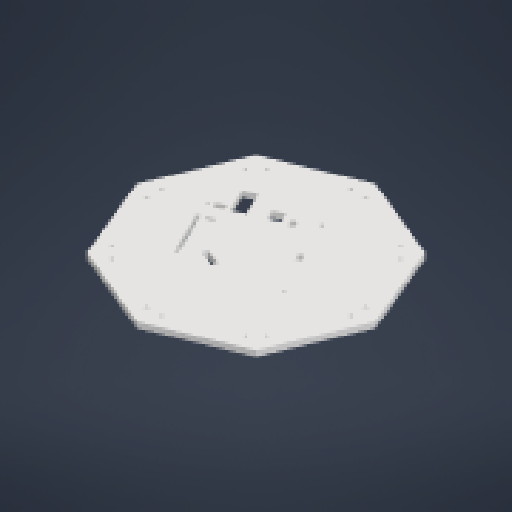
# Autodesk Inventor part: Bund
Saved by Autodesk Inventor 2026.1 (Build 301233020, 233B)
## iProperties
Created: 2026-04-22
Part Number: Bund
Material: Generic
Document SubType Name: Modeling
Designer: Mikke
Density: 1 g/cm^3
Appearance: Default
Author: Mikke
Autodesk Inventor part; units mm, degrees
ref_plane "YZ Plane" through (0, 0, 0) normal (1, 0, 0) x (0, 1, 0)
ref_plane "XZ Plane" through (0, 0, 0) normal (0, 1, 0) x (-1, 0, 0)
ref_plane "XY Plane" through (0, 0, 0) normal (0, 0, 1) x (1, 0, 0)
sketch "Sketch1" plane through (0, 0, 0) normal (0, 1, 0) x (-1, 0, 0)
  line L0 (0, 0) -> (0, -104.6)
  line L1 (0, -104.6) -> (-73.9634, -73.9634)
  line L2 (-73.9634, -73.9634) -> (-104.6, 0)
  line L3 (-104.6, 0) -> (-73.9634, 73.9634)
  line L4 (-73.9634, 73.9634) -> (0, 104.6)
  line L5 (0, 104.6) -> (73.9634, 73.9634)
  line L6 (73.9634, 73.9634) -> (104.6, 0)
  line L7 (104.6, 0) -> (73.9634, -73.9634)
  line L8 (73.9634, -73.9634) -> (0, -104.6)
  line L9 (89.2707, -89.2707) -> (126.2478, 0)
  line L10 (126.2478, 0) -> (89.2707, 89.2707)
  line L11 (89.2707, 89.2707) -> (0, 126.2478)
  line L12 (0, 126.2478) -> (-89.2707, 89.2707)
  line L13 (-89.2707, 89.2707) -> (-126.2478, 0)
  line L14 (-126.2478, 0) -> (-89.2707, -89.2707)
  line L15 (-89.2707, -89.2707) -> (0, -126.2478)
  line L16 (0, -126.2478) -> (89.2707, -89.2707)
  line L17 (0, -104.6) -> (7.6537, -123.0776)
  line L18 (0, -104.6) -> (20, -104.6) construction
  line L19 (73.9634, -73.9634) -> (81.617, -92.441)
  line L20 (73.9634, -73.9634) -> (76.2595, -79.5066)
  line L21 (76.2595, -79.5066) -> (70.7162, -81.8027)
  circle A0 centre (70.7162, -81.8027) radius 1.6
  line L22 (0, -104.6) -> (2.2961, -110.1433)
  line L23 (2.2961, -110.1433) -> (7.8394, -107.8472)
  circle A1 centre (7.8394, -107.8472) radius 1.6
  circle A2 centre (107.8472, -7.8394) radius 1.6
  circle A3 centre (81.8027, -70.7162) radius 1.6
  circle A4 centre (81.8027, 70.7162) radius 1.6
  circle A5 centre (107.8472, 7.8394) radius 1.6
  circle A6 centre (7.8394, 107.8472) radius 1.6
  circle A7 centre (70.7162, 81.8027) radius 1.6
  circle A8 centre (-70.7162, 81.8027) radius 1.6
  circle A9 centre (-7.8394, 107.8472) radius 1.6
  circle A10 centre (-107.8472, 7.8394) radius 1.6
  circle A11 centre (-81.8027, 70.7162) radius 1.6
  circle A12 centre (-81.8027, -70.7162) radius 1.6
  circle A13 centre (-107.8472, -7.8394) radius 1.6
  circle A14 centre (-7.8394, -107.8472) radius 1.6
  circle A15 centre (-70.7162, -81.8027) radius 1.6
  dimension "d0" = 104.6
  dimension "d1" = 20
  dimension "d2" = 67.5
  dimension "d3" = 6
  dimension "d4" = 6
  dimension "d5" = 3.2
  dimension "d6" = 6
  dimension "d7" = 3.2
  dimension "d10" = 360
  constraints: 48 end point, 16 centre point, 4 point on line, 3 coincident, 3 perpendicular, 1 equal length, 1 horizontal, 1 vertical, 57 other
  measures "d0" distance of L0.start L0.end
  measures "d1" distance between parallel lines of L7 L9
  measures "d2" angle of L17 L18
  measures "d3" distance of L7.end L20.end
  measures "d4" distance of L20.end L21.end
  measures "d5" diameter of A0
  measures "d6" distance of L22.end L23.end
  measures "d7" diameter of A1
extrude "Extrusion1" add sketch "Sketch1" along normal blind 6
sketch "Sketch2" plane through (0, 6, 0) normal (0, 1, 0) x (1, 0, 0)
  circle A0 centre (-42.6783, -41.3923) radius 1.25 projected
  circle A1 centre (-71.1016, 20.1286) radius 1.25 projected
  circle A2 centre (9.5684, 59.7961) radius 1.25 projected
  circle A3 centre (50.6037, -21.3711) radius 1.25 projected
  line L0 (27.326, 15.8388) -> (30.0184, 17.162) projected
  line L1 (30.0184, 17.162) -> (27.8131, 21.6494) projected
  line L2 (-6.9954, 48.8338) -> (-9.6878, 47.5107) projected
  line L3 (-9.6878, 47.5107) -> (-7.4825, 43.0233) projected
  line L4 (25.1207, 20.3262) -> (27.326, 15.8388) projected
  line L5 (27.8131, 21.6494) -> (25.1207, 20.3262) projected
  line L6 (-7.4825, 43.0233) -> (-4.7901, 44.3464) projected
  line L7 (-4.7901, 44.3464) -> (-6.9954, 48.8338) projected
  line L8 (-12.62, -33.9245) -> (-10.9955, -28.7261)
  line L9 (-10.9955, -28.7261) -> (-27.141, -23.6807)
  line L10 (-27.141, -23.6807) -> (-28.7655, -28.879)
  line L11 (-28.7655, -28.879) -> (-12.62, -33.9245)
  line L12 (-12.62, -33.9245) -> (-27.141, -23.6807) construction
  line L13 (-10.9955, -28.7261) -> (-28.7655, -28.879) construction
  line L14 (-45.832, -38.6971) -> (-42.9662, -37.2994)
  line L15 (-42.9662, -37.2994) -> (-63.3038, 4.3989)
  line L16 (-63.3038, 4.3989) -> (-66.1696, 3.0011)
  line L17 (-66.1696, 3.0011) -> (-45.832, -38.6971)
  line L18 (-45.832, -38.6971) -> (-63.3038, 4.3989) construction
  line L19 (-42.9662, -37.2994) -> (-66.1696, 3.0011) construction
  line L20 (-45.832, -38.6971) -> (-42.6435, -38.6971) construction
  line L21 (-57.8864, 3.7) -> (-59.1996, 6.4006)
  line L22 (-59.1996, 6.4006) -> (-52.2421, 9.7838)
  line L23 (-52.2421, 9.7838) -> (-50.9289, 7.0832)
  line L24 (-50.9289, 7.0832) -> (-57.8864, 3.7)
  line L25 (-64.7367, 19.4057) -> (-67.0188, 24.0494)
  line L26 (-67.0188, 24.0494) -> (-58.9321, 28.0235)
  line L27 (-58.9321, 28.0235) -> (-56.65, 23.3798)
  line L28 (-56.65, 23.3798) -> (-64.7367, 19.4057)
  line L29 (-52.2421, 24.5164) -> (-64.1558, 49.0938)
  line L30 (-64.1558, 49.0938) -> (-52.3886, 54.7979)
  line L31 (-52.3886, 54.7979) -> (-40.4749, 30.2205)
  line L32 (-40.4749, 30.2205) -> (-52.2421, 24.5164)
  line L33 (-29.4108, 46.112) -> (-24.4587, 36.7338)
  line L34 (-24.4587, 36.7338) -> (-14.7376, 41.867)
  line L35 (-14.7376, 41.867) -> (-19.6897, 51.2451)
  line L36 (-19.6897, 51.2451) -> (-29.4108, 46.112)
  circle A4 centre (9.5684, 59.7961) radius 1.75
  circle A5 centre (50.6037, -21.3711) radius 1.75
  circle A6 centre (-42.6783, -41.3923) radius 1.75
  circle A7 centre (-71.1016, 20.1286) radius 1.75
  line L37 (26.8696, 14.5003) -> (31.357, 16.7056)
  line L38 (31.357, 16.7056) -> (28.2696, 22.9879)
  line L39 (28.2696, 22.9879) -> (23.7822, 20.7827)
  line L40 (23.7822, 20.7827) -> (26.8696, 14.5003)
  line L41 (-6.539, 50.1724) -> (-11.0263, 47.9671)
  line L42 (-11.0263, 47.9671) -> (-7.9389, 41.6847)
  line L43 (-7.9389, 41.6847) -> (-3.4516, 43.89)
  line L44 (-3.4516, 43.89) -> (-6.539, 50.1724)
  point P0 (0, 0)
  point P1 (-19.8805, -28.8026)
  point P2 (-54.5679, -17.1491)
  dimension "d14" = 26
  dimension "d15" = 0.5
  dimension "d16" = 0.5
  dimension "d17" = 0.5
  dimension "d18" = 0.5
  dimension "d19" = 1
  dimension "d20" = 1
  constraints: 74 end point, 12 parallel, 6 perpendicular, 4 centre point, 4 midpoint, 1 equal length, 1 horizontal, 6 other
  measures "d14" angle of L20 L14
  measures "d15" radial gap between concentric circles of A2 A4
  measures "d16" radial gap between concentric circles of A3 A5
  measures "d17" radial gap between concentric circles of A0 A6
  measures "d18" radial gap between concentric circles of A1 A7
  measures "d19" distance between parallel lines of L4 L40
  measures "d20" distance between parallel lines of L7 L44
extrude "Extrusion2" cut sketch "Sketch2" against normal blind 7 contours A0 | A1 | A2 | A3 | L4 L5 L1 L0 | L7 L6 L3 L2 | L11 L10 L9 L8 | L17 L16 L15 L14 | L21 L22 L23 L24 | L25 L26 L27 L28 | L29 L30 L31 L32 | L36 L35 L34 L33 | A4 | A5 | A6 | A7 | L40 L39 L38 L37 | L44 L43 L42 L41
fillet "Fillet1" radius 2 8 edges at (89.2707, 3, 89.2707) (126.2478, 3, 0) (89.2707, 3, -89.2707) (0, 3, -126.2478) (-89.2707, 3, -89.2707) (-126.2478, 3, 0) (-89.2707, 3, 89.2707) (0, 3, 126.2478)
body "Solid1"
